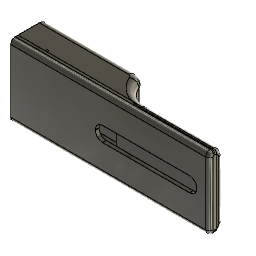
Model v1.0 (Autodesk Fusion 360 design; units mm, degrees)
Autodesk Fusion 360 part; units mm, degrees
sketch "Group 16 PCB" plane through (0, 0, 0) normal (0, 1, 0) x (1, 0, 0)
  circle A0 centre (50.5459, -63.6269) radius 0.4572
  circle A1 centre (-2.4131, -86.1059) radius 0.5105
  circle A2 centre (-10.668, -62.992) radius 0.762
  line L0 (78.9169, -56.2599) -> (78.9169, -90.2599)
  circle A3 centre (-14.097, -76.073) radius 0.762
  circle A4 centre (10.541, -64.135) radius 0.762
  circle A5 centre (46.8629, -63.4999) radius 0.4572
  circle A6 centre (21.5899, -78.6129) radius 0.4572
  line L1 (-1.5964, -82.7494) -> (-1.5964, -84.3826)
  circle A7 centre (7.0574, -79.6748) radius 0.65
  circle A8 centre (17.272, -59.182) radius 0.762
  circle A9 centre (-10.6681, -62.9919) radius 0.4572
  circle A10 centre (-3.0481, -60.0709) radius 0.508
  circle A11 centre (10.5409, -64.1349) radius 0.4572
  circle A12 centre (-7.8741, -73.5329) radius 0.4572
  circle A13 centre (7.0574, -82.2148) radius 0.65
  arc A14 (28.065, -64.006) -> (28.065, -65.026) centre (28.065, -64.516) ccw
  circle A15 centre (11.4299, -76.0729) radius 0.4572
  line L2 (-12.2682, -61.0108) -> (-14.1478, -61.0108)
  circle A16 centre (16.764, -67.691) radius 0.762
  circle A17 centre (-2.4131, -83.5659) radius 0.5105
  circle A18 centre (-13.2081, -60.0709) radius 0.508
  circle A19 centre (14.8589, -67.8179) radius 0.4572
  circle A20 centre (-5.588, -60.071) radius 0.9398
  circle A21 centre (14.859, -67.818) radius 0.762
  circle A22 centre (7.4384, -77.008) radius 0.762
  circle A23 centre (12.8994, -85.136) radius 0.762
  line L3 (8.0075, -81.265) -> (8.0075, -83.165)
  circle A24 centre (-6.3501, -76.5809) radius 0.4572
  circle A25 centre (16.891, -60.96) radius 0.762
  circle A26 centre (7.0574, -79.675) radius 0.95
  circle A27 centre (8.255, -69.469) radius 0.762
  circle A28 centre (-8.1281, -60.0709) radius 0.5639
  circle A29 centre (8.382, -61.595) radius 0.762
  circle A30 centre (21.5899, -69.5959) radius 0.4572
  line L4 (-14.1478, -61.0108) -> (-14.1478, -59.1312)
  arc A31 (-16.634, -64.006) -> (-16.634, -65.026) centre (-16.634, -64.516) ccw
  line L5 (8.0075, -83.165) -> (6.1075, -83.165)
  circle A32 centre (-9.0171, -65.1509) radius 0.4572
  circle A33 centre (-0.508, -60.071) radius 0.9398
  circle A34 centre (8.3819, -61.5949) radius 0.4572
  line L6 (27.065, -63.516) -> (27.065, -65.516)
  circle A35 centre (16.7639, -67.6909) radius 0.4572
  circle A36 centre (-17.145, -85.09) radius 0.762
  circle A37 centre (75.3097, -86.2317) radius 0.8
  circle A38 centre (6.4769, -63.7539) radius 0.4572
  circle A39 centre (3.429, -75.565) radius 0.762
  line L7 (-21.0831, -56.2599) -> (78.9169, -56.2599)
  circle A40 centre (-4.9531, -83.5659) radius 0.5105
  circle A41 centre (11.43, -76.073) radius 0.762
  circle A42 centre (21.3359, -67.3099) radius 0.4572
  circle A43 centre (10.5409, -66.6749) radius 0.4572
  circle A44 centre (-4.953, -83.566) radius 0.8166
  line L8 (-3.2296, -82.7494) -> (-1.5964, -82.7494)
  circle A45 centre (-10.6681, -60.0709) radius 0.508
  line L9 (78.9169, -90.2599) -> (-21.0831, -90.2599)
  circle A46 centre (-14.0971, -76.0729) radius 0.4572
  arc A47 (28.065, -65.026) -> (28.065, -64.006) centre (28.065, -64.516) ccw
  circle A48 centre (11.938, -58.42) radius 0.762
  circle A49 centre (8.2549, -69.4689) radius 0.4572
  circle A50 centre (-9.017, -65.151) radius 0.762
  circle A51 centre (-8.128, -60.071) radius 0.9398
  circle A52 centre (3.1749, -63.7539) radius 0.4572
  line L10 (-12.2682, -59.1312) -> (-12.2682, -61.0108)
  circle A53 centre (-7.493, -86.106) radius 0.8166
  circle A54 centre (-10.668, -60.071) radius 0.9398
  circle A55 centre (3.175, -63.754) radius 0.762
  circle A56 centre (-7.493, -83.566) radius 0.8166
  circle A57 centre (-5.5881, -60.0709) radius 0.508
  circle A58 centre (21.59, -69.596) radius 0.762
  circle A59 centre (-6.35, -76.581) radius 0.762
  line L11 (29.065, -65.516) -> (29.065, -63.516)
  circle A60 centre (-18.542, -73.261) radius 0.8
  circle A61 centre (10.541, -66.675) radius 0.762
  circle A62 centre (12.8994, -85.1358) radius 0.4572
  circle A63 centre (17.2719, -59.1819) radius 0.4572
  circle A64 centre (-16.635, -64.516) radius 1
  circle A65 centre (11.9379, -58.4199) radius 0.4572
  circle A66 centre (1.905, -69.469) radius 0.762
  circle A67 centre (-7.874, -73.533) radius 0.762
  line L12 (-21.0831, -90.2599) -> (-21.0831, -56.2599)
  circle A68 centre (-13.843, -68.961) radius 0.762
  circle A69 centre (46.863, -63.5) radius 0.762
  circle A70 centre (3.4289, -75.5649) radius 0.4572
  circle A71 centre (50.546, -63.627) radius 0.762
  circle A72 centre (-3.048, -60.071) radius 0.9398
  line L13 (-14.1478, -59.1312) -> (-12.2682, -59.1312)
  circle A73 centre (-7.4931, -86.1059) radius 0.5105
  circle A74 centre (-0.5081, -60.0709) radius 0.508
  circle A75 centre (6.477, -63.754) radius 0.762
  circle A76 centre (7.4384, -77.0078) radius 0.4572
  line L14 (29.065, -63.516) -> (27.065, -63.516)
  line L15 (-3.2296, -84.3826) -> (-3.2296, -82.7494)
  line L16 (27.065, -65.516) -> (29.065, -65.516)
  circle A77 centre (21.336, -67.31) radius 0.762
  circle A78 centre (-13.8431, -68.9609) radius 0.4572
  circle A79 centre (1.9049, -69.4689) radius 0.4572
  line L17 (-1.5964, -84.3826) -> (-3.2296, -84.3826)
  circle A80 centre (-2.413, -86.106) radius 0.8166
  circle A81 centre (-7.4931, -83.5659) radius 0.5105
  circle A82 centre (-17.1451, -85.0899) radius 0.4572
  circle A83 centre (-3.302, -79.629) radius 0.762
  circle A84 centre (16.8909, -60.9599) radius 0.4572
  circle A85 centre (-4.9531, -86.1059) radius 0.5105
  line L18 (6.1075, -81.265) -> (8.0075, -81.265)
  circle A86 centre (75.3097, -60.2318) radius 0.8
  line L19 (6.1075, -83.165) -> (6.1075, -81.265)
  circle A87 centre (-4.953, -86.106) radius 0.8166
  circle A88 centre (21.59, -78.613) radius 0.762
  circle A89 centre (-3.3021, -79.6289) radius 0.4572
  arc A90 (-16.634, -65.026) -> (-16.634, -64.006) centre (-16.634, -64.516) ccw
sketch "Sketch1" plane through (0, 0, 0) normal (0, 1, 0) x (1, 0, 0) in component "case"
  line L0 (-21.0831, -56.2599) -> (78.9169, -56.2599) construction
  line L1 (78.9169, -56.2599) -> (78.9169, -90.2599) construction
  line L2 (78.9169, -90.2599) -> (-21.0831, -90.2599) construction
  line L3 (-21.0831, -90.2599) -> (-21.0831, -56.2599) construction
  line L4 (-22.0831, -55.2599) -> (79.9169, -55.2599) construction
  line L5 (79.9169, -55.2599) -> (79.9169, -91.2599) construction
  line L6 (79.9169, -91.2599) -> (-22.0831, -91.2599) construction
  line L7 (-22.0831, -91.2599) -> (-22.0831, -55.2599) construction
  line L8 (-24.0831, -53.2599) -> (81.9169, -53.2599)
  line L9 (81.9169, -93.2599) -> (-24.0831, -93.2599)
  line L10 (-24.0831, -93.2599) -> (-24.0831, -53.2599)
  line L11 (-16.634, -64.516) -> (-17.779, -64.516) construction
  line L12 (28.065, -64.516) -> (29.21, -64.516) construction
  line L13 (29.21, -64.516) -> (29.21, -91.2599) construction
  line L14 (81.9169, -93.2599) -> (85.9169, -93.2599)
  line L15 (81.9169, -53.2599) -> (85.9169, -53.2599)
  line L16 (85.9169, -53.2599) -> (85.9169, -93.2599)
  line L17 (29.21, -87.7446) -> (41.91, -87.7446) construction
  line L18 (41.91, -87.7446) -> (41.91, -53.2599)
  line L19 (41.91, -87.7446) -> (41.91, -93.2599)
  line L20 (81.9169, -93.2599) -> (81.9169, -53.2599)
  line L21 (29.21, -89.0097) -> (31.21, -89.0097) construction
  line L22 (31.21, -89.0097) -> (31.21, -53.2599)
  line L23 (31.21, -89.0097) -> (31.21, -93.2599)
  circle A0 centre (75.3097, -86.2317) radius 0.8
  circle A1 centre (75.3097, -60.2318) radius 0.8
  line L24 (79.9169, -73.2599) -> (78.9169, -73.2599) construction
  line L25 (78.9169, -73.2599) -> (78.9169, -77.3599) construction
  line L26 (78.9169, -77.3599) -> (22.7799, -77.3599)
  line L27 (22.7799, -77.3599) -> (22.7799, -69.1599)
  line L28 (22.7799, -69.1599) -> (78.9169, -69.1599)
  line L29 (78.9169, -69.1599) -> (78.9169, -77.3599)
  circle A2 centre (-18.542, -73.261) radius 0.8
  point P0 (-21.0831, -56.2599)
  point P1 (78.9169, -90.2599)
  point P2 (-16.634, -64.516)
  point P3 (28.065, -64.516)
  point P4 (75.3097, -86.2317)
  point P5 (75.3097, -60.2318)
  dimension "d1" = -1
  dimension "d3" = 1.145
  dimension "d4" = 1.145
  dimension "d5" = 4
  dimension "d6" = 4
  dimension "d7" = 12.7
  dimension "d13" = 2
  dimension "d36" = 4.1
  dimension "d37" = 56.137
  dimension "d38" = 8.2
  constraint horizontal L0
  constraint vertical L1
  constraint horizontal L2
  constraint vertical L3
  constraint coincident P1 L1.end
  constraint coincident P0 L0.start
  constraint coincident P2 L11.start
  constraint horizontal L11
  constraint coincident P3 L12.start
  constraint horizontal L12
  constraint coincident L6 L13.end
  constraint perpendicular L6 L13
  constraint parallel L0 L8
  constraint parallel L2 L9
  constraint parallel L3 L10
  constraint parallel L9 L14
  constraint parallel L8 L15
  constraint perpendicular L14 L16
  constraint coincident L13 L17.start
  constraint perpendicular L13 L17
  constraint coincident L8 L18.end
  constraint perpendicular L8 L18
  constraint coincident L9 L19.end
  constraint perpendicular L9 L19
  constraint coincident L13 L21.start
  constraint perpendicular L13 L21
  constraint coincident L8 L22.end
  constraint perpendicular L8 L22
  constraint coincident L9 L23.end
  constraint perpendicular L9 L23
  constraint midpoint L5 L24.start
  constraint midpoint L1 L24.end
  constraint perpendicular L24 L25
  constraint horizontal L26
  constraint vertical L27
  constraint horizontal L28
  constraint vertical L29
  measures "d3" distance of P2 L11.end
  measures "d4" distance of P3 L12.end
  measures "d5" distance of L9.start L14.end
  measures "d6" distance of L8.end L15.end
  measures "d7" distance of L17.start L17.end
  measures "d13" distance of L21.start L21.end
  measures "d36" distance of L24.end L25.end
  measures "d37" distance of L25.end L26.end
  measures "d38" distance of L25.end L28.end
extrude "Extrude3" add sketch "Sketch1" along normal blind 19.8 contours L8 L9 L10 L22 L23 L26 L27 L28 | L22 L26 L27 L28 | A2 makes body 1 in component "case"
shell "Shell3" thickness 2 removed faces 0 bodies 1 in component "case"
extrude "Extrude5" add sketch "Sketch1" along normal blind 7.1 contours L8 L18 L22 L28 | L8 L9 L18 L19 L20 L26 L28 L29 | L18 L22 L26 L28 | L9 L18 L19 L22 L23 L26 | L18 L26 L28 L29 | A0 | A1 bodies 1 in component "case"
sketch "Sketch2" plane through (81.9169, 0, 0) normal (1, 0, 0) x (0, 1, 0) in component "case"
  line L0 (0, 93.2599) -> (0, 53.2599)
  line L1 (0, 53.2599) -> (7.1, 53.2599)
  line L2 (7.1, 53.2599) -> (7.1, 93.2599)
  line L3 (7.1, 93.2599) -> (0, 93.2599)
  line L4 (2, 55.2599) -> (5.1, 55.2599)
  line L5 (5.1, 55.2599) -> (5.1, 91.2599)
  line L6 (5.1, 91.2599) -> (2, 91.2599)
  line L7 (2, 91.2599) -> (2, 55.2599)
  dimension "d22" = -2
extrude "Extrude6" cut sketch "Sketch2" against normal blind 60 from surface at -2 contours L4 L5 L6 L7 bodies 1 in component "case"
extrude "Extrude7" add sketch "Sketch1" along normal blind 7.1 contours L14 L15 L16 L20 bodies 1 in component "case"
fillet "Fillet1" radius 6 1 edges at (31.21, 19.8, 73.2599) on bodies 1 in component "case"
fillet "Fillet2" radius 15 1 edges at (31.21, 7.1, 73.2599) on bodies 1 in component "case"
fillet "Fillet3" radius 4 8 edges at (65.2085, 7.1, 93.2599) (36.2517, 9.5715, 93.2599) (28.5093, 18.8114, 93.2599) (0.5634, 19.8, 93.2599) (65.2085, 7.1, 53.2599) (36.2517, 9.5715, 53.2599) (28.5093, 18.8114, 53.2599) (0.5634, 19.8, 53.2599) on bodies 1 in component "case"
fillet "Fillet4" radius 2.5 2 edges at (30.9169, 0, 93.2599) (30.9169, 0, 53.2599) on bodies 1 in component "case"
fillet "Fillet5" radius 2 8 edges at (85.9169, 2.8, 53.2599) (85.9169, 0.7322, 53.9921) (85.9169, 0, 73.2599) (85.9169, 0.7322, 92.5276) (85.9169, 2.8, 93.2599) (85.9169, 5.9284, 92.0883) (85.9169, 7.1, 73.2599) (85.9169, 5.9284, 54.4315) on bodies 1 in component "case"
extrude "Extrude8" cut sketch "Group 16 PCB" along normal blind 6.5 from surface at 1 contours A37 | A86 bodies 1 in component "case"
thread "Thread1" "ISO Metric profile 1.6 M1.6x0.35 6H" major diameter 1.668 minor diameter 1.271 pitch 0.35 angle 60 modelled right hand crest width 0.0916 on face at (75.4486, 5.7667, 59.4439) crest through (75.9452, 5.1875, 60.2318) on bodies 1 in component "case"
thread "Thread2" "ISO Metric profile 1.6 M1.6x0.35 6H" major diameter 1.668 minor diameter 1.271 pitch 0.35 angle 60 modelled right hand crest width 0.0916 on face at (75.4486, 1.3333, 59.4439) crest through (75.9452, 1.0875, 60.2318) on bodies 1 in component "case"
thread "Thread3" "ISO Metric profile 1.6 M1.6x0.35 6H" major diameter 1.668 minor diameter 1.271 pitch 0.35 angle 60 modelled right hand crest width 0.0916 on face at (75.4486, 5.7667, 85.4439) crest through (75.9452, 5.1875, 86.2317) on bodies 1 in component "case"
thread "Thread4" "ISO Metric profile 1.6 M1.6x0.35 6H" major diameter 1.668 minor diameter 1.271 pitch 0.35 angle 60 modelled right hand crest width 0.0916 on face at (75.4486, 1.3333, 85.4439) crest through (75.9452, 1.0875, 86.2317) on bodies 1 in component "case"
extrude "Extrude9" cut sketch "Sketch1" along normal blind 2.2 contours L18 L22 L26 L28 | L22 L26 L27 L28 | L18 L26 L28 L29 bodies 1 in component "case"
ref_plane "WorkPlane1" through (30.9169, 9.9, 53.2599) normal (0, 0, -1) x (-1, 0, 0) in component "case"
sketch "Sketch3" plane through (29.9169, 9.15, 53.2599) normal (0, 0, -1) x (1, 0, 0) in component "case"
  line L0 (54, 9) -> (54, 5) construction
  dimension "d42" = 4
  constraint vertical L0
  measures "d42" distance of L0.start L0.end
ref_plane "WorkPlane2" through (61.9134, 4, 73.2599) normal (0, 1, 0) x (1, 0, 0) in component "case"
split "Split1" by plane through (61.9134, 4, 73.2599) normal (0, 1, 0) bodies 1 makes body 2 at (11.9272, 17.8, 79.2599) in component "case"
fillet "Fillet6" radius 4 4 edges at (22.7799, 1, 69.1599) (22.7799, 1, 77.3599) (78.9169, 1, 77.3599) (78.9169, 1, 69.1599) on bodies 1 in component "case"
extrude "Extrude10" add sketch "Sketch1" along normal blind 4.5 separate body contours A2 makes body 3 in component "case"
sketch "Sketch4" plane through (0, 0, 93.2599) normal (0, 0, 1) x (-1, 0, 0) in component "case"
  line L0 (-38.7217, -4) -> (24.0831, -4)
  line L1 (24.0831, -4) -> (24.0831, -2.5)
  line L2 (24.0831, -2.5) -> (-83.9169, -2.5)
  line L3 (-83.9169, -2.5) -> (-83.9169, -3.1)
  line L4 (-83.9169, -3.1) -> (-44.5001, -3.1)
  arc A0 (-38.7217, -4) -> (-44.5001, -3.1) centre (-44.5001, -22.1) ccw
  line L5 (24.0831, -4) -> (9.0831, -4) construction
  line L6 (9.0831, -4) -> (9.0831, -5.5)
  line L7 (9.0831, -5.5) -> (8, -5)
  line L8 (8, -5) -> (8.2411, -4.4777)
  line L9 (8.2411, -4.4777) -> (8.2411, -4)
  line L10 (9.0831, -4) -> (8.2411, -4)
  dimension "d47" = 15
  dimension "d48" = 1.5
  constraint coincident L0.end L1.start
  constraint perpendicular L1 L5
  constraint perpendicular L5 L6
  constraint perpendicular L7 L8
  constraint coincident L0 L9.end
  constraint perpendicular L0 L9
  measures "d47" distance of L0.end L5.end
  measures "d48" distance of L5.end L6.end
extrude "Extrude11" add sketch "Sketch4" against normal blind 2 contours L0 L6 L7 L8 L9 L10 bodies 1 in component "case"
ref_plane "WorkPlane3" through (29.9169, 4, 73.2599) normal (0, 0, 1) x (1, 0, 0) in component "case"
sketch "Sketch5" plane through (0, 0, 53.2599) normal (0, 0, -1) x (1, 0, 0) in component "case"
  line L0 (-24.0831, -4) -> (38.7217, -4)
  arc A0 (44.5001, -3.1) -> (38.7217, -4) centre (44.5001, -22.1) ccw
  line L1 (44.5001, -3.1) -> (83.9169, -3.1)
  line L2 (83.9169, -3.1) -> (83.9169, -2.5)
  line L3 (83.9169, -2.5) -> (-24.0831, -2.5)
  line L4 (-24.0831, -2.5) -> (-24.0831, -4)
  line L5 (-9.0831, -4) -> (-9.0831, -5.5)
  line L6 (-9.0831, -5.5) -> (-8, -5)
  line L7 (-8, -5) -> (-8.2411, -4.4777)
  line L8 (-8.2411, -4.4777) -> (-8.2411, -4)
  point P0 (-9.0831, -5.5)
  point P1 (-8, -5)
  point P2 (-8.2411, -4.4777)
  point P3 (-8.2411, -4)
  point P4 (-9.0831, -4)
  constraint coincident P4 L5.start
  constraint coincident P0 L5.end
  constraint coincident P1 L6.end
  constraint coincident P2 L7.end
  constraint coincident P3 L8.end
extrude "Extrude12" add sketch "Sketch5" against normal blind 2 contours L0 L5 L6 L7 L8 bodies 1 in component "case"
fillet "Fillet7" radius 0.3 2 edges at (-9.0831, 5.5, 54.2599) (-9.0831, 5.5, 92.2599) on bodies 1 in component "case"
fillet "Fillet8" radius 0.3 4 edges at (-8, 5, 92.2599) (-8.2411, 4.4777, 92.2599) (-8, 5, 54.2599) (-8.2411, 4.4777, 54.2599) on bodies 1 in component "case"
combine "Combine1" operation add target body 3 tool bodies 1 in component "case"
combine "Combine2" operation cut target body 2 tool bodies 3 keep tools in component "case"
extrude "Extrude1" [suppressed] in component "case"
shell "Shell1" [suppressed] in component "case"
extrude "Extrude2" [suppressed] in component "case"
shell "Shell2" [suppressed] in component "case"
extrude "Extrude4" [suppressed] in component "case"
component "case" placed x (1, 0, 0) y (0, 1, 0) z (0, 0, 1) at (0, 0, 0)
named bodies: "Top", "Bottom"
